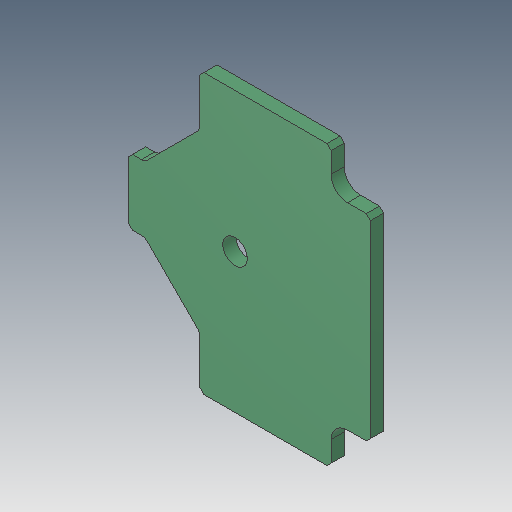
# Autodesk Inventor part: force_sensor_pcb
Saved by Autodesk Inventor 2019.4 (Build 234330000, 330)
## iProperties
Created: 2018-10-05
Part Number: force_sensor_pcb
Material: 一般
Document SubType Name: Modeling
Designer: student
Density: 1 g/cm^3
Appearance: 滑らか - 濃い海緑
Mass: 1.22766 g
Surface Area: 17.3353 cm^2
Volume: 1.22766 cm^3
Author: student
Autodesk Inventor part; units mm, degrees
ref_plane "YZ Plane" through (0, 0, 0) normal (1, 0, 0) x (0, 1, 0)
ref_plane "XZ Plane" through (0, 0, 0) normal (0, 1, 0) x (-1, 0, 0)
ref_plane "XY Plane" through (0, 0, 0) normal (0, 0, 1) x (1, 0, 0)
sketch "スケッチ1" plane through (0, 0, 0) normal (0, 0, 1) x (1, 0, 0)
  line L0 (16.5, 0) -> (16.5, 11.5)
  line L1 (11.2044, 17) -> (-3.7956, 17)
  line L2 (-3.7956, 17) -> (-4.2956, 16.5)
  line L3 (-4.2956, 16.5) -> (-4.2956, 11.1093)
  arc A0 (-4.5885, 10.4022) -> (-4.2956, 11.1093) centre (-5.2956, 11.1093) ccw
  line L4 (-4.5885, 10.4022) -> (-10.6978, 4.2929)
  arc A1 (-11.4049, 4) -> (-10.6978, 4.2929) centre (-11.4049, 5) ccw
  line L5 (-11.4049, 4) -> (-12.5, 4)
  line L6 (-12.5, 4) -> (-13, 3.5)
  line L7 (-13, 3.5) -> (-13, 0)
  circle A2 centre (0, 0) radius 1.5
  line L8 (16, 12) -> (13.7044, 12)
  line L9 (11.7044, 14) -> (11.7044, 16.5)
  line L10 (16.5, 11.5) -> (16, 12)
  line L11 (11.7044, 16.5) -> (11.2044, 17)
  line L12 (0, 0) -> (16.5, 0) construction
  arc A3 (11.7044, 14) -> (13.7044, 12) centre (13.7044, 14) ccw
  line L13 (11.7044, 17) -> (11.7044, 18.5) construction
  line L14 (0, 0) -> (-13, 0) construction
  line L15 (-13, -2) -> (-13, 2) construction
  line L16 (-10.6978, 4.2929) -> (-5.2974, 9.6932) construction
  line L17 (-4.2956, 17) -> (-4.2956, 11.1093) construction
  line L18 (16.5, 0) -> (16.5, -11.5)
  line L19 (11.2044, -17) -> (-3.7956, -17)
  line L20 (-3.7956, -17) -> (-4.2956, -16.5)
  line L21 (-4.2956, -16.5) -> (-4.2956, -11.1093)
  arc A4 (-4.2956, -11.1093) -> (-4.5885, -10.4022) centre (-5.2956, -11.1093) ccw
  line L22 (-4.5885, -10.4022) -> (-10.6978, -4.2929)
  arc A5 (-10.6978, -4.2929) -> (-11.4049, -4) centre (-11.4049, -5) ccw
  line L23 (-11.4049, -4) -> (-12.5, -4)
  line L24 (-12.5, -4) -> (-13, -3.5)
  line L25 (-13, -3.5) -> (-13, 0)
  line L26 (16, -12) -> (13.7044, -12)
  line L27 (11.7044, -14) -> (11.7044, -16.5)
  line L28 (16.5, -11.5) -> (16, -12)
  line L29 (11.7044, -16.5) -> (11.2044, -17)
  arc A6 (13.7044, -12) -> (11.7044, -14) centre (13.7044, -14) ccw
  dimension "d5" = 0.5
  dimension "d6" = 0.5
  dimension "d7" = 16.5
  dimension "d8" = 2
  dimension "d9" = 12
  dimension "d10" = 17
  dimension "d11" = 0.5
  dimension "d12" = 0.5
  dimension "d14" = 0.5
  dimension "d15" = 0.5
  dimension "d16" = 4
  dimension "d18" = 0.5
  dimension "d19" = 0.5
  dimension "d20" = 1
  dimension "d21" = 3
  constraints: 52 end point, 17 symmetric about line, 12 point on circle, 7 centre point, 6 tangent, 4 collinear, 3 horizontal, 2 perpendicular, 1 coincident, 1 equal radius, 1 vertical, 3 other
  measures "d5" distance from line of L0.end L8
  measures "d6" distance from line of L8.start L0
  measures "d7" distance from line of L0 L12.start
  measures "d8" radius of A3
  measures "d9" distance between parallel lines of L12 L8
  measures "d10" distance between parallel lines of L12 L1
  measures "d11" distance from line of L9.end L1
  measures "d12" distance from line of L1.start L9
  measures "d14" distance from line of L5 L6.end
  measures "d15" distance from line of L5.end L7
  measures "d16" distance between parallel lines of L12 L5
  measures "d18" distance from line of L1.end L3
  measures "d19" distance from line of L2.end L1
  measures "d20" radius of A1
  measures "d21" diameter of A2
extrude "押し出し1" add sketch "スケッチ1" along normal blind 1.6
